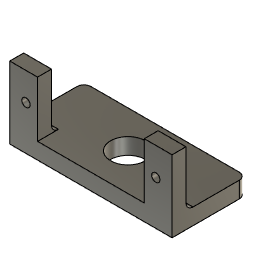
FirstPassArmv12 (Autodesk Fusion 360 archive; units mm, degrees)
design "Arm1_flange"
Autodesk Fusion 360 part; units mm, degrees
sketch "Sketch1" plane through (0, 0, 0) normal (0, 0, 1) x (1, 0, 0)
  line L0 (0, 0) -> (-35, 0)
  line L1 (-35, 0) -> (-35, 16)
  line L2 (-35, 16) -> (0, 16)
  line L3 (0, 16) -> (0, 0)
  dimension "d14" = 16
  dimension "d15" = 35
  constraint horizontal L0
  constraint vertical L1
  constraint horizontal L2
  constraint vertical L3
  constraint coincident L0.start L3.end
  measures "d14" distance of L0.end L1.end
  measures "d15" distance of L1.end L2.end
extrude "Extrude1" add sketch "Sketch1" along normal blind 3.5
sketch "Sketch3" plane through (0, 0, 0) normal (0, 1, 0) x (1, 0, 0)
  line L0 (0, -3.5) -> (-6, -3.5)
  line L1 (-6, -3.5) -> (-6, -15.5)
  line L2 (-6, -15.5) -> (0, -15.5)
  line L3 (0, -15.5) -> (0, -3.5)
  line L4 (-35, -3.5) -> (-29, -3.5)
  line L5 (-29, -3.5) -> (-29, -15.5)
  line L6 (-29, -15.5) -> (-35, -15.5)
  line L7 (-35, -15.5) -> (-35, -3.5)
  point P0 (0, -3.5)
  point P1 (-35, -3.5)
  dimension "d17" = 12
  dimension "d19" = 23
  constraint horizontal L0
  constraint vertical L1
  constraint horizontal L2
  constraint vertical L3
  constraint horizontal L4
  constraint vertical L5
  constraint horizontal L6
  constraint vertical L7
  constraint equal L2 L6
  constraint equal L3 L5
  constraint coincident P0 L0.start
  constraint horizontal L1.end L5.end
  constraint coincident P1 L4.start
  measures "d17" distance of P0 L2.end
  measures "d19" distance of L1 L5
extrude "Extrude3" add sketch "Sketch3" along normal blind 3
sketch "Sketch4" plane through (0, 0, 3.5) normal (0, 0, 1) x (-1, 0, 0)
  line L0 (6, 0) -> (6, -3)
  line L1 (6, -3) -> (0, -3)
  line L2 (0, -3) -> (0, -16)
  line L3 (0, -16) -> (35, -16)
  line L4 (35, -16) -> (35, -3)
  line L5 (35, -3) -> (29, -3)
  line L6 (29, -3) -> (29, 0)
  line L7 (29, 0) -> (6, 0)
  line L8 (0, -16) -> (35, 0) construction
  line L9 (35, -16) -> (0, 0) construction
  circle A0 centre (17.5, -8) radius 3.75
  dimension "d22" = 7.5
  constraint coincident L2.end L3.start
  constraint coincident L3.end L4.start
  constraint coincident L9.end origin
  constraint midpoint L9 A0.centre
  measures "d22" diameter of A0
extrude "Extrude4" cut sketch "Sketch4" against normal up to surface (3.5 mm away) contours A0
sketch "Sketch7" plane through (0, 3, 0) normal (0, 1, 0) x (-1, 0, 0)
  line L0 (0, 15.5) -> (0, 3.5)
  line L1 (0, 3.5) -> (6, 3.5)
  line L2 (6, 3.5) -> (6, 15.5)
  line L3 (6, 15.5) -> (0, 15.5)
  line L4 (0, 9.5) -> (35, 9.5) construction
  line L5 (35, 3.5) -> (35, 15.5) construction
  circle A0 centre (3.5, 9.5) radius 0.9
  circle A1 centre (31.5, 9.5) radius 0.9
  line L6 (32.4, 9.5) -> (32.3186, 9.874) construction
  point P0 (17.5, 9.5)
  dimension "d30" = 1.8
  dimension "d31" = 14
  dimension "d32" = 1.8
  dimension "d33" = 14
  constraint midpoint L0 L4.start
  constraint perpendicular L0 L4
  constraint coincident L4.end L5
  constraint coincident L4 A0.centre
  constraint midpoint L4 P0
  constraint coincident L4 A1.centre
  constraint coincident A1 L6.start
  constraint coincident L4 L6.start
  constraint coincident A1 L6.end
  measures "d30" diameter of A0
  measures "d31" distance of A0.centre P0
  measures "d32" diameter of A1
  measures "d33" distance of P0 A1.centre
extrude "Extrude6" cut sketch "Sketch7" against normal up to surface (3 mm away) contours A0 | A1
fillet "Fillet1" radius 1.5 2 edges at (-3, 3, 3.5) (-32, 3, 3.5)
fillet "Fillet2" radius 1.5 2 edges at (0, 16, 1.75) (-35, 16, 1.75)
extrude "Extrude2" [suppressed]
hole "Hole1" [suppressed]
hole "Hole2" [suppressed]
hole "Hole3" [suppressed]
